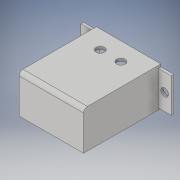
# Autodesk Inventor part: Caixa do sensor de temperatura
Saved by Autodesk Inventor 2019 (Build 230136000, 136)
## iProperties
Created: 2020-05-31
Part Number: Caixa do sensor de temperatura
Material: Genérico
Document SubType Name: Modeling
Designer: Público
Density: 1 g/cm^3
Appearance: Padrão
Author: Público
Autodesk Inventor part; units mm, degrees
ref_plane "YZ Plane" through (0, 0, 0) normal (1, 0, 0) x (0, 1, 0)
ref_plane "XZ Plane" through (0, 0, 0) normal (0, 1, 0) x (-1, 0, 0)
ref_plane "XY Plane" through (0, 0, 0) normal (0, 0, 1) x (1, 0, 0)
sketch "Esboço1" plane through (0, 0, 0) normal (0, 1, 0) x (-1, 0, 0)
  line L0 (0, 0) -> (25, 0)
  line L1 (25, 0) -> (25, -30)
  line L2 (25, -30) -> (0, -30)
  line L3 (0, -30) -> (0, 0)
  dimension "d0" = 25
  dimension "d1" = 30
  constraints: 8 end point, 2 parallel, 1 horizontal, 1 perpendicular
  measures "d0" distance of L1.end L2.end
  measures "d1" distance of L0.end L1.end
extrude "Extrusão1" add sketch "Esboço1" along normal blind 15
shell "Casca1" thickness 1 removed faces 1 at (-8.3333, 15, -10)
sketch "Esboço4" plane through (-24, 1, -1) normal (0, 1, 0) x (1, 0, 0)
  line L0 (24, 29) -> (-1, 29) projected
  line L1 (-1, 29) -> (-1, -1) projected
  circle A0 centre (11.5, 14.5) radius 3.5
  point P0 (24, -1)
  point P1 (1, 29)
  dimension "d17" = 7
  dimension "d20" = 12.5
  dimension "d21" = 14.5
  constraints: 1 centre point
  measures "d17" diameter of A0
  measures "d20" distance from line of L1 A0.centre
  measures "d21" distance from line of L0 A0.centre
extrude "Extrusão4" cut sketch "Esboço4" against normal blind 5
sketch "Esboço10" plane through (0, 0, 0) normal (0, -1, 0) x (1, 0, 0)
  circle A0 centre (-12.5, -15.5) radius 3.5 projected
  circle A1 centre (-16.5, -23) radius 1.65
  circle A2 centre (-8.5, -23) radius 1.65
  point P0 (0, 0)
  dimension "d72" = 3.3
  dimension "d73" = 3.3
  dimension "d113" = 7.5
  dimension "d114" = 4
  constraints: 2 centre point, 1 coincident
  measures "d72" diameter of A1
  measures "d73" diameter of A2
  measures "d113" vertical distance of A2.centre A0.centre
  measures "d114" horizontal distance of point (-12.5, -15.5) A2.centre
extrude "Extrusão10" cut sketch "Esboço10" against normal blind 10 contours A1 | A2
sketch "Esboço11" plane through (0, 0, -30) normal (0, 0, -1) x (-1, 0, 0)
  line L0 (1, 1) -> (1, 15) projected
  line L1 (24, 1) -> (24, 15) projected
  line L2 (1, 1) -> (24, 1)
  line L3 (24, 1) -> (24, 14)
  line L4 (24, 14) -> (1, 14)
  line L5 (1, 14) -> (1, 1)
  line L6 (0, 15) -> (25, 15) projected
  point P0 (0, 0)
  dimension "d80" = 1
  constraints: 8 end point, 2 parallel, 1 horizontal, 1 perpendicular, 1 point on line
  measures "d80" distance between parallel lines of L6 L4
extrude "Extrusão11" cut sketch "Esboço11" against normal blind 10 contours L0 L4 L1 L2
sketch "Esboço12" plane through (-1, 1, -1) normal (0, 0, -1) x (-1, 0, 0)
  line L0 (0, 13) -> (0, 14) projected
  line L1 (0, 14) -> (23, 14)
  line L2 (23, 14) -> (23, 13)
  line L3 (23, 13) -> (0, 13)
  line L4 (0, 13) -> (0, 14)
  point P0 (-1, -1)
  constraints: 8 end point, 2 parallel, 1 horizontal, 1 perpendicular
extrude "Extrusão12" add sketch "Esboço12" along normal up to surface (28 mm away)
sketch "Esboço13" plane through (0, 0, 0) normal (0, -1, 0) x (1, 0, 0)
  circle A0 centre (-16.5, -23) radius 1.65 projected
  circle A1 centre (-16.5, -23) radius 1.65
  circle A2 centre (-8.5, -23) radius 1.65 projected
  circle A3 centre (-8.5, -23) radius 1.65
  point P0 (0, 0)
  constraints: 2 centre point, 2 coincident
extrude "Extrusão13" cut sketch "Esboço13" against normal up to surface (15 mm away)
sketch "Esboço14" plane through (0, 0, -30) normal (0, 0, -1) x (-1, 0, 0)
  line L0 (0, 0.7381) -> (-5, 0.7381)
  line L1 (-5, 0.7381) -> (-5, 14)
  line L2 (-5, 14) -> (0, 14)
  line L3 (0, 14) -> (0, 0.7381)
  line L4 (1, 14) -> (24, 14) projected
  line L5 (25, 0) -> (25, 15) projected
  line L6 (25, 1) -> (30, 1)
  line L7 (30, 1) -> (30, 14)
  line L8 (30, 14) -> (25, 14)
  line L9 (25, 14) -> (25, 1)
  line L10 (24, 1) -> (1, 1) projected
  point P0 (0, 0)
  dimension "d88" = 5
  dimension "d89" = 0
  dimension "d90" = 5
  dimension "d91" = 0
  dimension "d92" = 0
  constraints: 16 end point, 4 parallel, 2 horizontal, 2 perpendicular, 1 point on line
  measures "d88" distance between parallel lines of L3 L1
  measures "d89" distance between parallel lines of L4 L2
  measures "d90" distance of L8.end L7.end
  measures "d91" distance between parallel lines of L4 L8
  measures "d92" distance between parallel lines of L10 L6
extrude "Extrusão14" add sketch "Esboço14" against normal blind 1
sketch "Esboço15" plane through (0, 0, -30) normal (0, 0, -1) x (-1, 0, 0)
  circle A0 centre (27.5, 7.5) radius 1.5
  circle A1 centre (-2.5, 7.2381) radius 1.5
  line L0 (25, 1) -> (30, 1) projected
  line L1 (0, 0.7381) -> (-5, 0.7381) projected
  line L2 (-5, 0.7381) -> (-5, 14) projected
  line L3 (30, 1) -> (30, 14) projected
  point P0 (0, 0)
  dimension "d95" = 3
  dimension "d96" = 3
  dimension "d97" = 6.5
  dimension "d98" = 6.5
  dimension "d99" = 2.5
  dimension "d100" = 2.5
  constraints: 2 centre point
  measures "d95" diameter of A0
  measures "d96" diameter of A1
  measures "d97" distance from line of L0 A0.centre
  measures "d98" distance from line of L1 A1.centre
  measures "d99" distance from line of L2 A1.centre
  measures "d100" distance from line of L3 A0.centre
extrude "Extrusão15" cut sketch "Esboço15" against normal blind 1
fillet "Arredondamento4" radius 1.5 1 edges at (-12.5, 15, 0)
